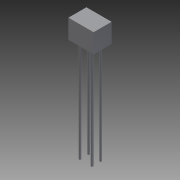
# Autodesk Inventor part: LineSensor
Saved by Autodesk Inventor 2011 SP2 (Build 150309200, 309)
## iProperties
Created: 2015-01-25
Part Number: LineSensor
Document SubType Name: Modeling
Designer: Ernest
Density: 1 g/cm^3
Mass: 0.146817 g
Surface Area: 3.1037 cm^2
Volume: 0.146817 cm^3
Author: Ernest
Autodesk Inventor part; units mm, degrees
ref_plane "YZ Plane" through (0, 0, 0) normal (1, 0, 0) x (0, 1, 0)
ref_plane "XZ Plane" through (0, 0, 0) normal (0, 1, 0) x (-1, 0, 0)
ref_plane "XY Plane" through (0, 0, 0) normal (0, 0, 1) x (1, 0, 0)
sketch "Sketch1" plane through (0, 0, 0) normal (0, 0, 1) x (1, 0, 0)
  line L0 (0, 0) -> (6.15, 0)
  line L1 (6.15, 0) -> (6.15, 4.4)
  line L2 (6.15, 4.4) -> (0, 4.4)
  line L3 (0, 4.4) -> (0, 0)
  dimension "d0" = 6.15
  dimension "d1" = 4.4
  constraints: 8 end point, 2 parallel, 1 horizontal, 1 perpendicular
  measures "d0" distance of L2.end L1.end
  measures "d1" distance of L0.end L1.end
extrude "Extrusion1" add sketch "Sketch1" against normal blind 4.7
sketch "Sketch2" plane through (0, 0, -4.7) normal (0, 0, -1) x (-1, 0, 0)
  line L0 (-6.15, 0) -> (-6.15, 4.4) projected
  line L1 (0, 4.4) -> (0, 0) projected
  line L2 (-6.15, 4.4) -> (0, 4.4) projected
  circle A0 centre (-4.545, 3.353) radius 0.25
  circle A1 centre (-1.605, 3.353) radius 0.25
  circle A2 centre (-4.545, 1.253) radius 0.25
  circle A3 centre (-1.605, 1.253) radius 0.25
  dimension "d4" = 0.5
  dimension "d5" = 0.5
  dimension "d6" = 0.5
  dimension "d7" = 0.5
  dimension "d8" = 3.44
  dimension "d9" = 3.44
  dimension "d10" = 2.6
  dimension "d11" = 2.6
  dimension "d12" = 1.605
  dimension "d13" = 1.605
  dimension "d14" = 1.605
  dimension "d15" = 1.047
  constraints: 4 centre point
  measures "d4" diameter of A0
  measures "d5" diameter of A2
  measures "d6" diameter of A1
  measures "d7" diameter of A3
  measures "d12" distance from line of L1 A1.centre
  measures "d13" distance from line of L0 A0.centre
  measures "d14" distance from line of L0 A2.centre
  measures "d15" distance from line of L2 A1.centre
extrude "Extrusion2" add sketch "Sketch2" along normal blind 25
body "Solid1"
